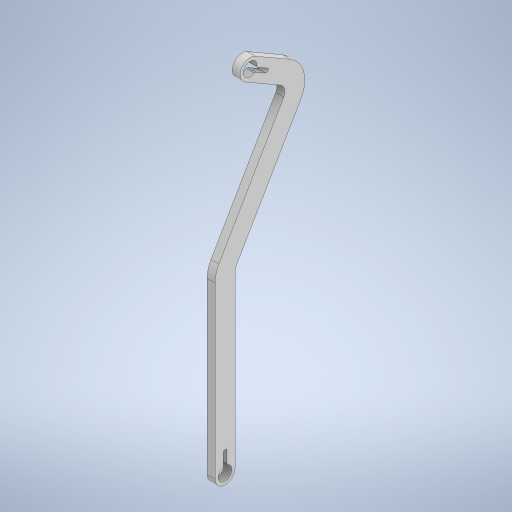
# Autodesk Inventor part: Door Upper Parallel Bar
Saved by Autodesk Inventor 2024 (Build 280153000, 153)
## iProperties
Created: 2024-08-28
Part Number: Door Upper Parallel Bar
Material: Generic
Document SubType Name: Modeling
Designer: Ishaan
Density: 1 g/cm^3
Appearance: Default
Author: Ishaan
Autodesk Inventor part; units mm, degrees
ref_plane "YZ Plane" through (0, 0, 0) normal (1, 0, 0) x (0, 1, 0)
ref_plane "XZ Plane" through (0, 0, 0) normal (0, 1, 0) x (-1, 0, 0)
ref_plane "XY Plane" through (0, 0, 0) normal (0, 0, 1) x (1, 0, 0)
sketch "Sketch1" plane through (0, 0, 0) normal (1, 0, 0) x (0, 1, 0)
  line L0 (-10, -10) -> (10, -10) construction
  line L1 (10, -10) -> (10, 10) construction
  line L2 (10, 10) -> (-10, 10) construction
  line L3 (-10, 10) -> (-10, -10) construction
  line L4 (-10, -10) -> (10, 10) construction
  line L5 (10, -10) -> (-10, 10) construction
  line L6 (0, 0) -> (135.9808, 0)
  line L7 (253.6603, -48.3013) -> (270, -20)
  line L8 (114.9075, -11.5) -> (119.815, -20) construction
  line L9 (119.815, -20) -> (114.9075, -28.5) construction
  line L10 (114.9075, -28.5) -> (105.0925, -28.5) construction
  line L11 (105.0925, -28.5) -> (100.185, -20) construction
  line L12 (100.185, -20) -> (105.0925, -11.5) construction
  line L13 (105.0925, -11.5) -> (114.9075, -11.5) construction
  line L14 (143.4808, -2.0096) -> (233.1699, -53.7917)
  arc A0 (233.1699, -53.7917) -> (253.6603, -48.3013) centre (240.6699, -40.8013) ccw
  arc A1 (143.4808, -2.0096) -> (135.9808, 0) centre (135.9808, -15) ccw
  point P0 (140, 0)
  point P1 (246.1603, -61.2917)
  point P2 (110, -20)
  dimension "d0" = 270
  dimension "d4" = 20
  dimension "d5" = 20
  dimension "d60" = 20
  dimension "d65" = 17
  dimension "d66" = 160
  dimension "d68" = 11.5
  dimension "d82" = 150
  dimension "d83" = 140
  dimension "d84" = 15
  dimension "d93" = 15
  constraints: 30 end point, 4 point on circle, 4 point on line, 4 tangent, 3 perpendicular, 2 centre point, 2 horizontal, 2 midpoint, 2 parallel, 1 coincident, 1 horizontal alignment, 13 other
  measures "d0" horizontal distance of point (0, 0) L7.end
  measures "d4" distance of L2.end L1.end
  measures "d5" distance of L1.end L0.end
  measures "d60" vertical distance of point (0, 0) L7.end
  measures "d65" distance between parallel lines of L10 L13
  measures "d66" distance of L7.end point (110, -20)
  measures "d68" distance between parallel lines of L13 L6
  measures "d82" angle of L14 L6
  measures "d83" distance of point (0, 0) point (140, 0)
  measures "d84" radius of A0
  measures "d93" radius of A1
surface extrude "ExtrusionSrf1" sketch "Sketch1" along normal mid plane 6.35 shown no curves L6 A1 L14 A0 L7
thicken "Thicken1" operation new thickness 16 both sides yes extend neighbours no toward (0, 0, 1) faces at (-1.0583, 45.3269, 0) (1.0583, 139.44, -0.4043) (1.0583, 173.3771, -19.2703) (1.0583, 244.0077, -55.4252) (-1.0583, 259.1068, -38.8675)
sketch "Sketch4" plane through (3.175, 0, 8) normal (1, 0, 0) x (0, 0, -1)
  line L0 (60.3013, 260.5885) -> (32, 276.9282) projected
  line L1 (32, 276.9282) -> (24, 263.0718) projected
  line L2 (52.3013, 246.7321) -> (24, 263.0718) projected
  arc A0 (54.8634, 237.1699) -> (52.3013, 246.7321) centre (48.8013, 240.6699) ccw projected
  line L3 (3.0814, 147.4808) -> (54.8634, 237.1699) projected
  line L4 (0, 0) -> (0, 135.9808) projected
  line L5 (16, 0) -> (0, 0) projected
  line L6 (16, 0) -> (16, 135.9808) projected
  line L7 (16.9378, 139.4808) -> (68.7199, 229.1699) projected
  arc A1 (68.7199, 229.1699) -> (60.3013, 260.5885) centre (48.8013, 240.6699) ccw projected
  line L8 (16, 0) -> (0, 0) projected
  circle A2 centre (8, 0) radius 8
  circle A3 centre (28, 270) radius 8
  arc A4 (3.0814, 147.4808) -> (0, 135.9808) centre (23, 135.9808) ccw projected
  arc A5 (16.9378, 139.4808) -> (16, 135.9808) centre (23, 135.9808) ccw projected
  constraints: 2 coincident, 2 midpoint, 1 horizontal alignment, 5 other
extrude "Extrusion2" add sketch "Sketch4" against normal up to surface (6.35 mm away) contours L1 A3 | A2 L5 | L5 A2 picked at (25.5467, 271.0452)
hole "Hole4" at (3.175, 0, 0) at (3.175, 270, -20) direction (-1, 0, 0) diameter 11.05 end through all
sketch "Sketch5" plane through (3.175, 0, 0) normal (1, 0, 0) x (0, 0, -1)
  line L0 (-8, 0) -> (-8, 135.9808) projected
  arc A0 (-8, 0) -> (8, 0) centre (0, 0) ccw projected
  line L1 (8, 0) -> (8, 135.9808) projected
  line L2 (8.9378, 139.4808) -> (60.7199, 229.1699) projected
  arc A1 (60.7199, 229.1699) -> (52.3013, 260.5885) centre (40.8013, 240.6699) ccw projected
  line L3 (52.3013, 260.5885) -> (24, 276.9282) projected
  arc A2 (24, 276.9282) -> (16, 263.0718) centre (20, 270) ccw projected
  line L4 (44.3013, 246.7321) -> (16, 263.0718) projected
  arc A3 (46.8634, 237.1699) -> (44.3013, 246.7321) centre (40.8013, 240.6699) ccw projected
  line L5 (-4.9186, 147.4808) -> (46.8634, 237.1699) projected
  circle A4 centre (0, 0) radius 5.525 projected
  circle A5 centre (20, 270) radius 5.525 projected
  line L6 (20, 270) -> (32.9904, 262.5) construction
  line L7 (19.25, 268.701) -> (32.2404, 261.201)
  line L8 (33.7404, 263.799) -> (20.75, 271.299)
  arc A6 (20.75, 271.299) -> (19.25, 268.701) centre (20, 270) ccw
  arc A7 (32.2404, 261.201) -> (33.7404, 263.799) centre (32.9904, 262.5) ccw
  line L9 (0, 0) -> (0, 15) construction
  line L10 (1.5, 0) -> (1.5, 15)
  line L11 (-1.5, 15) -> (-1.5, 0)
  arc A8 (-1.5, 0) -> (1.5, 0) centre (0, 0) ccw
  arc A9 (1.5, 15) -> (-1.5, 15) centre (0, 15) ccw
  arc A10 (8.9378, 139.4808) -> (8, 135.9808) centre (15, 135.9808) ccw projected
  arc A11 (-4.9186, 147.4808) -> (-8, 135.9808) centre (15, 135.9808) ccw projected
  point P0 (0, 0)
  point P1 (26.4952, 266.25)
  point P2 (0, 7.5)
  point P3 (-1.5, 5.3175)
  point P4 (1.5, 5.3175)
  point P5 (25.3551, 268.6403)
  point P6 (23.8551, 266.0422)
  dimension "d86" = 3
  dimension "d87" = 15
  constraints: 16 end point, 8 point on circle, 8 tangent, 4 centre point, 3 parallel, 2 midpoint, 1 equal length, 1 equal radius, 1 vertical
  measures "d86" diameter of A7
  measures "d87" distance of L6.start L6.end
extrude "Extrusion3" cut sketch "Sketch5" against normal through all contours A4 L11 A9 L10 | A5 L8 A7 L7
fillet "Fillet4" radius 1 4 edges at (0, 266.0422, -23.8551) (0, 268.6403, -25.3551) (0, 5.3175, 1.5) (0, 5.3175, -1.5)
body "Solid1"
body "Srf1"
